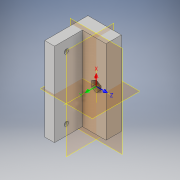
# Autodesk Inventor part: cam_holder_hog_part
Saved by Autodesk Inventor 2019 (Build 230136000, 136)
## iProperties
Created: 2024-08-06
Part Number: cam_holder_hog_part
Material: Generisch
Document SubType Name: Modeling
Designer: nic
Density: 1 g/cm^3
Appearance: Vorgabe
Author: nic
Autodesk Inventor part; units mm, degrees
ref_plane "YZ Plane" through (0, 0, 0) normal (1, 0, 0) x (0, 1, 0)
ref_plane "XZ Plane" through (0, 0, 0) normal (0, 1, 0) x (-1, 0, 0)
ref_plane "XY Plane" through (0, 0, 0) normal (0, 0, 1) x (1, 0, 0)
sketch "Skizze1" plane through (0, 0, 0) normal (0, 0, 1) x (1, 0, 0)
  line L0 (-13.5, 30) -> (13.5, 30)
  line L1 (13.5, 30) -> (13.5, -30)
  line L2 (13.5, -30) -> (-13.5, -30)
  line L3 (-13.5, -30) -> (-13.5, 30)
  line L4 (-13.5, 30) -> (13.5, -30) construction
  line L5 (13.5, 30) -> (-13.5, -30) construction
  point P0 (0, 0)
  dimension "d0" = 27
  dimension "d1" = 60
  constraints: 12 end point, 2 midpoint, 2 parallel, 1 horizontal, 1 perpendicular
  measures "d0" distance of L1.end L2.end
  measures "d1" distance of L0.end L1.end
extrude "Extrusion1" add sketch "Skizze1" along normal blind 11
sketch "Skizze2" plane through (0, 0, 11) normal (0, 0, 1) x (1, 0, 0)
  line L0 (13.5, 30) -> (-13.5, 30) projected
  line L1 (-13.5, -30) -> (13.5, -30) projected
  line L2 (-13.5, 30) -> (-3.5, 30)
  line L3 (-3.5, 30) -> (-3.5, -30)
  line L4 (-3.5, -30) -> (-13.5, -30)
  line L5 (-13.5, -30) -> (-13.5, 30)
  point P0 (0, 0)
  dimension "d4" = 10
  constraints: 8 end point, 2 parallel, 1 horizontal, 1 perpendicular, 1 point on line
  measures "d4" distance of L3.end L4.end
extrude "Extrusion2" add sketch "Skizze2" along normal blind 20
sketch "Skizze3" plane through (-3.5, -30, 11) normal (1, 0, 0) x (0, 0, -1)
  line L0 (0, 60) -> (0, 0) construction
  line L1 (0, 60) -> (-20, 60) construction
  line L2 (-20, 0) -> (-20, 60) construction
  line L3 (0, 0) -> (-20, 0) construction
  line L4 (0, 60) -> (0, 0) projected
  line L5 (0, 30) -> (-11.5, 30) construction
  line L6 (-11.5, 30) -> (-11.5, 52.5) construction
  line L7 (-11.5, 30) -> (-11.5, 7.5) construction
  circle A0 centre (-11.5, 7.5) radius 1.55
  circle A1 centre (-11.5, 52.5) radius 1.55
  point P0 (11, 30)
  dimension "d7" = 11.5
  dimension "d8" = 22.5
  dimension "d9" = 22.5
  dimension "d10" = 3.1
  dimension "d11" = 3.1
  constraints: 6 end point, 2 centre point, 2 coincident, 2 vertical, 1 horizontal, 1 midpoint
  measures "d7" distance of L5.start L5.end
  measures "d8" distance of L5.end L6.end
  measures "d9" distance of L5.end L7.end
  measures "d10" diameter of A0
  measures "d11" diameter of A1
extrude "Extrusion3" cut sketch "Skizze3" against normal through all
sketch "Skizze4" plane through (-13.5, -30, 0) normal (-1, 0, 0) x (0, 0, 1)
  circle A0 centre (22.5, 7.5) radius 1.55 projected
  circle A1 centre (22.5, 52.5) radius 1.55 projected
  line L0 (0, 0) -> (0, 60) projected
  line L1 (0, 0) -> (31, 0) projected
  line L2 (31, 60) -> (31, 0) projected
  line L3 (0, 60) -> (31, 60) projected
  point P0 (0, 30)
extrude "Extrusion4" cut sketch "Skizze4" against normal blind 3
sketch "Skizze5" plane through (-10.5, -30, 0) normal (-1, 0, 0) x (0, 0, 1)
  line L0 (-3, 30.25) -> (3, 30.25)
  line L1 (3, 30.25) -> (3, 29.75)
  line L2 (3, 29.75) -> (-3, 29.75)
  line L3 (-3, 29.75) -> (-3, 30.25)
  line L4 (-3, 30.25) -> (3, 29.75) construction
  line L5 (3, 30.25) -> (-3, 29.75) construction
  point P0 (0, 30)
  dimension "d16" = 6
  dimension "d17" = 0.5
  constraints: 12 end point, 2 midpoint, 2 parallel, 1 horizontal, 1 perpendicular
  measures "d16" distance of L1.end L2.end
  measures "d17" distance of L0.end L1.end
extrude "Extrusion5" cut sketch "Skizze5" against normal blind 0.5
sketch "Skizze6" plane through (0, 0, 11) normal (0, 0, 1) x (1, 0, 0)
  line L0 (-3.5, -30) -> (-3.5, 30) projected
  line L1 (-3.5, 0) -> (6.5, 0)
  circle A0 centre (6.5, 0) radius 2.05
  point P0 (0, 0)
  dimension "d20" = 10
  dimension "d21" = 4.1
  constraints: 2 end point, 1 centre point, 1 coincident, 1 horizontal, 1 midpoint
  measures "d20" distance of L1.start L1.end
  measures "d21" diameter of A0
extrude "Extrusion6" cut sketch "Skizze6" against normal through all
sketch "Skizze7" plane through (0, 0, 11) normal (0, 0, 1) x (1, 0, 0)
  circle A0 centre (6.5, 0) radius 2.05 projected
  line L0 (6.5, 0) -> (6.5, 4)
  line L1 (6.5, 0) -> (14.5, 0) construction
  line L2 (6.5, 4) -> (9.9641, 2)
  line L3 (9.9641, 2) -> (9.9641, -2)
  line L4 (9.9641, -2) -> (6.5, -4)
  line L5 (6.5, -4) -> (3.0359, -2)
  line L6 (3.0359, -2) -> (3.0359, 2)
  line L7 (3.0359, 2) -> (6.5, 4)
  point P0 (0, 0)
  dimension "d24" = 4
  constraints: 16 end point, 1 coincident, 1 horizontal, 1 vertical, 13 other
  measures "d24" distance of L0.start L0.end
extrude "Extrusion7" cut sketch "Skizze7" against normal blind 4
ref_plane "Arbeitsebene1" through (6.5, 0, 11) normal (0, 0, 1) x (1, 0, 0)
ref_plane "Arbeitsebene2" through (6.5, 0, 11) normal (0, 1, 0) x (1, 0, 0)
ref_plane "Arbeitsebene3" through (6.5, 0, 11) normal (1, 0, 0) x (0, 0, -1)
